cobalt robot blade_v4 (Autodesk Fusion 360 design; units mm, degrees)
Autodesk Fusion 360 part; units mm, degrees
sketch "center" plane through (0, 0, 0) normal (0, 0, 1) x (1, 0, 0)
  line L0 (3.9767, 19.6007) -> (11, 21)
  line L1 (11, 21) -> (9.3026, 17.7049)
  arc A0 (3.9767, 19.6007) -> (0, 20) centre (0, 0) ccw
  arc A1 (11.8706, 16.0962) -> (9.3026, 17.7049) centre (0, 0) ccw
  arc A2 (-8.3037, 18.1947) -> (-11.7557, 16.1803) centre (0, 0) ccw
  line L2 (-8.3037, 18.1947) -> (-3.4443, 23.455)
  line L3 (-3.4443, 23.455) -> (-2.8807, 19.7915)
  arc A3 (0.1424, 19.9995) -> (-2.8807, 19.7915) centre (0, 0) ccw
  arc A4 (-17.4124, 9.839) -> (-19.0211, 6.1803) centre (0, 0) ccw
  line L4 (-17.4124, 9.839) -> (-16.573, 16.951)
  line L5 (-16.573, 16.951) -> (-13.9637, 14.3184)
  arc A5 (-11.6402, 16.2636) -> (-13.9637, 14.3184) centre (0, 0) ccw
  arc A6 (-19.8702, -2.2748) -> (-19.0211, -6.1803) centre (0, 0) ccw
  line L6 (-19.8702, -2.2748) -> (-23.3714, 3.9723)
  line L7 (-23.3714, 3.9723) -> (-19.713, 3.3762)
  arc A7 (-18.9766, 6.3156) -> (-19.713, 3.3762) centre (0, 0) ccw
  arc A8 (-14.7382, -13.5198) -> (-11.7557, -16.1803) centre (0, 0) ccw
  line L8 (-14.7382, -13.5198) -> (-21.2427, -10.5237)
  line L9 (-21.2427, -10.5237) -> (-17.9326, -8.8556)
  arc A9 (-19.0647, -6.0447) -> (-17.9326, -8.8556) centre (0, 0) ccw
  arc A10 (-3.9767, -19.6007) -> (0, -20) centre (0, 0) ccw
  line L10 (-3.9767, -19.6007) -> (-11, -21)
  line L11 (-11, -21) -> (-9.3026, -17.7049)
  arc A11 (-11.8706, -16.0962) -> (-9.3026, -17.7049) centre (0, 0) ccw
  arc A12 (8.3037, -18.1947) -> (11.7557, -16.1803) centre (0, 0) ccw
  line L12 (8.3037, -18.1947) -> (3.4443, -23.455)
  line L13 (3.4443, -23.455) -> (2.8807, -19.7915)
  arc A13 (-0.1424, -19.9995) -> (2.8807, -19.7915) centre (0, 0) ccw
  arc A14 (17.4124, -9.839) -> (19.0211, -6.1803) centre (0, 0) ccw
  line L14 (17.4124, -9.839) -> (16.573, -16.951)
  line L15 (16.573, -16.951) -> (13.9637, -14.3184)
  arc A15 (11.6402, -16.2636) -> (13.9637, -14.3184) centre (0, 0) ccw
  arc A16 (19.8702, 2.2748) -> (19.0211, 6.1803) centre (0, 0) ccw
  line L16 (19.8702, 2.2748) -> (23.3714, -3.9723)
  line L17 (23.3714, -3.9723) -> (19.713, -3.3762)
  arc A17 (18.9766, -6.3156) -> (19.713, -3.3762) centre (0, 0) ccw
  arc A18 (14.7382, 13.5198) -> (11.7557, 16.1803) centre (0, 0) ccw
  line L18 (14.7382, 13.5198) -> (21.2427, 10.5237)
  line L19 (21.2427, 10.5237) -> (17.9326, 8.8556)
  arc A19 (19.0647, 6.0447) -> (17.9326, 8.8556) centre (0, 0) ccw
  circle A20 centre (0, 0) radius 2.75
  dimension "d248" = 40
  dimension "d250" = 360
  dimension "d253" = 5.5
  constraint coincident A0.centre A1.centre
  constraint coincident A1.start A0
  constraint concentric A0 A1
  constraint concentric A7 A20
  measures "d248" diameter of A0
  measures "d253" diameter of A20
extrude "Extrude13" add sketch "center" along normal blind 4
equation "d = 4 mm"
equation "StockHeight = 3 mm"
equation "d250 = 360.0 °"
